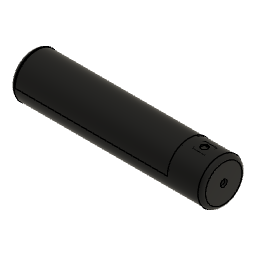
Laser_Pointer_Assembled (Autodesk Fusion 360 archive; units mm, degrees)
design "Laser_Pointer_Case"
Autodesk Fusion 360 part; units mm, degrees
sketch "Sketch1" plane through (0, 0, 0) normal (1, 0, 0) x (0, 1, 0)
  circle A0 centre (0, 0) radius 9.5
  circle A1 centre (0, 0) radius 11.5
  dimension "d1" = 19
  dimension "d2" = 23
  constraint coincident A0.centre A1.centre
  measures "d1" diameter of A0
  measures "d2" diameter of A1
extrude "Extrude1" add sketch "Sketch1" along normal blind 50 makes body 1
extrude "Extrude2" add 1 faces at (0, 10.7551, -1.0433) along direction (-1, 0, 0) blind 50 on bodies 1 bodies 1
sketch "Sketch3" plane through (-50, 0, 0) normal (-1, 0, 0) x (0, -1, 0)
  circle A0 centre (0, 0) radius 9.5
  circle A1 centre (0, 0) radius 11.5
extrude "Extrude4" add sketch "Sketch3" against normal blind 5 contours A0 bodies 1
ref_plane "WorkPlane1" through (0, 0, -11.5) normal (0, 0, 1) x (1, 0, 0)
sketch "Sketch2" plane through (0, 0, -11.5) normal (0, 0, 1) x (1, 0, 0)
  line L0 (-45, -15.7965) -> (35, -15.7965)
  line L1 (35, -15.7965) -> (35, 17.9404)
  line L2 (35, 17.9404) -> (-45, 17.9404)
  line L3 (-45, 17.9404) -> (-45, -15.7965)
  circle A0 through (-50, 11.5, 11.5) (-50, -5.75, 21.4593) (-50, -5.75, 1.5407)
  point P0 (-50, 0)
  dimension "d8" = 80
  dimension "d16" = 5
  constraint horizontal L0
  constraint vertical L1
  constraint horizontal L2
  constraint vertical L3
  measures "d8" distance of L0.start L0.end
  measures "d16" distance of L3 P0
extrude "Extrude3" cut sketch "Sketch2" along normal blind 11.5 bodies 1
sketch "Sketch4" plane through (35, 0, 0) normal (-1, 0, 0) x (0, -1, 0)
  arc A0 (-9.5, 0) -> (9.5, 0) centre (0, 0) ccw
  line L0 (-9.5, 0) -> (-11.5, 0)
  arc A1 (-11.5, 0) -> (11.5, 0) centre (0, 0) ccw
  line L1 (11.5, 0) -> (9.5, 0)
  circle A2 centre (0, 0) radius 9.5
  dimension "d13" = 19
  constraint coincident A0.centre A1.centre
  measures "d13" diameter of A2
extrude "Extrude5" add sketch "Sketch4" against normal blind 2 contours A0 A2 bodies 1
sketch "Sketch5" plane through (-45, 0, 0) normal (1, 0, 0) x (0, 1, 0)
  arc A0 (9.5, 0) -> (-9.5, 0) centre (0, 0) ccw
  line L0 (-9.5, 0) -> (-11.5, 0)
  arc A1 (-11.5, 0) -> (11.5, 0) centre (0, 0) ccw
  line L1 (11.5, 0) -> (9.5, 0)
  circle A2 centre (0, 0) radius 9.5
  dimension "d17" = 19
  constraint coincident A0.centre A1.centre
  measures "d17" diameter of A2
extrude "Extrude6" add sketch "Sketch5" along normal blind 80 separate body contours L0 A1 L1 A2 makes body 2
extrude "Extrude7" cut 1 faces at (-45, -0.2865, -3.8226) along direction (-1, 0, 0) blind 2.5 on bodies 1 bodies 1
extrude "Extrude8" add 1 faces at (-45, 10.5848, -2.1732) along direction (-1, 0, 0) blind 2.5 on bodies 2 bodies 2
sketch "Sketch6" plane through (-47.5, 0, 0) normal (-1, 0, 0) x (0, -1, 0)
  line L0 (11.5, 0) -> (9.5, 0)
  arc A0 (-9.5, 0) -> (9.5, 0) centre (0, 0) ccw
  line L1 (-9.5, 0) -> (-11.5, 0)
  arc A1 (-11.5, 0) -> (11.5, 0) centre (0, 0) ccw
  circle A2 centre (0, 0) radius 9.5
  dimension "d24" = 19
  constraint concentric A0 A2
  measures "d24" diameter of A2
extrude "Extrude9" add sketch "Sketch6" against normal blind 2.5 contours A0 A2 bodies 2
sketch "Sketch7" plane through (-50, 0, 0) normal (-1, 0, 0) x (0, -1, 0)
  circle A0 centre (0, 0) radius 11.5
  circle A1 centre (0, 0) radius 1.25
  dimension "d27" = 2.5
  constraint concentric A0 A1
  measures "d27" diameter of A1
extrude "Extrude10" cut sketch "Sketch7" against normal blind 5 contours A1 bodies 1 2
ref_plane "WorkPlane2" through (-39.5, 0, -1) normal (1, 0, 0) x (0, 1, 0)
sketch "Sketch8" plane through (-39.5, 0, 0) normal (1, 0, 0) x (0, 1, 0)
  circle A0 centre (0, 0) radius 9.5
  dimension "d31" = 19
  constraint coincident A0.centre origin
  measures "d31" diameter of A0
extrude "Extrude11" add sketch "Sketch8" along normal blind 2 bodies 1
sketch "Sketch9" plane through (35, 0, 0) normal (-1, 0, 0) x (0, -1, 0)
  line L0 (-9.5, 0) -> (-11.5, 0)
  arc A0 (-11.5, 0) -> (11.5, 0) centre (0, 0) ccw
  line L1 (11.5, 0) -> (9.5, 0)
  arc A1 (9.5, 0) -> (-9.5, 0) centre (0, 0) ccw
  circle A2 centre (0, 0) radius 2.5
  dimension "d34" = 5
  constraint coincident A0.centre A1.centre
  measures "d34" diameter of A2
extrude "Extrude12" cut sketch "Sketch9" against normal blind 2 contours A2 bodies 1
sketch "Sketch10" plane through (-37.5, 0, 0) normal (1, 0, 0) x (0, 1, 0)
  arc A0 (-9.5, 0) -> (9.5, 0) centre (0, 0) ccw
  arc A1 (9.5, 0) -> (-9.5, 0) centre (0, 0) ccw
  circle A2 centre (0, 0) radius 2.5
  dimension "d37" = 5
  constraint coincident A0.centre A1.centre
  measures "d37" diameter of A2
extrude "Extrude13" cut sketch "Sketch10" against normal blind 2 contours A2 bodies 1
extrude "Extrude14" add 1 faces at (35, -7.3712, -2.0248) along direction (-1, 0, 0) blind 3 on bodies 1 bodies 1
extrude "Extrude15" cut 1 faces at (37, 7.122, 0.5962) along direction (-1, 0, 0) blind 4 on bodies 1 bodies 1
extrude "Extrude16" cut 1 faces at (50, 10.7551, -1.0433) along direction (-1, 0, 0) blind 2 on bodies 1 bodies 1
sketch "Sketch11" plane through (48, 0, 0) normal (1, 0, 0) x (0, 1, 0)
  circle A0 centre (0, 0) radius 9.5
  circle A1 centre (0, 0) radius 11.5
  circle A2 centre (0, 0) radius 11.5
  dimension "d46" = 23
  constraint concentric A0 A2
  measures "d46" diameter of A2
extrude "Extrude17" add sketch "Sketch11" along normal blind 2 separate body contours A0 | A1 A2 makes body 3
sketch "Sketch12" plane through (50, 0, 0) normal (1, 0, 0) x (0, 1, 0)
  circle A0 centre (0, 0) radius 11.5
  circle A1 centre (0, 0) radius 1.75
  dimension "d49" = 3.5
  constraint coincident A0.centre A1.centre
  measures "d49" diameter of A1
extrude "Extrude18" cut sketch "Sketch12" against normal blind 2 contours A1 bodies 3
sketch "Sketch13" plane through (48, 0, 0) normal (1, 0, 0) x (0, 1, 0)
  circle A0 centre (0, 0) radius 9.5
  circle A1 centre (0, 0) radius 11.5
  circle A2 centre (0, 0) radius 10.875
  circle A3 centre (0, 0) radius 10.125
  circle A4 centre (0, 0) radius 10.925
  circle A5 centre (0, 0) radius 10.075
  dimension "d52" = 21.75
  dimension "d53" = 20.25
  dimension "d54" = 0.05
  dimension "d55" = -0.05
  constraint concentric A0 A2
  constraint concentric A0 A3
  measures "d52" diameter of A2
  measures "d53" diameter of A3
extrude "Extrude19" cut sketch "Sketch13" against normal blind 3 contours A2 | A3 | A4 bodies 1
sketch "Sketch14" plane through (48, 0, 0) normal (-1, 0, 0) x (0, -1, 0)
  circle A0 centre (0, 0) radius 1.75
  circle A1 centre (0, 0) radius 11.5
  circle A2 centre (0, -0.0586) radius 3
  circle A3 centre (0, -0.0586) radius 3.2
  circle A4 centre (0, 0) radius 10.925
  circle A5 centre (0, 0) radius 10.075
  circle A6 centre (0, 0) radius 10.875
  circle A7 centre (0, 0) radius 10.125
  dimension "d58" = 0.2
  dimension "d61" = -0.05
  dimension "d62" = 0.05
extrude "Extrude20" cut sketch "Sketch14" against normal blind 0.75 contours A2 | A3 bodies 3
extrude "Extrude21" add sketch "Sketch14" along normal blind 2.9 contours A6 bodies 3
ref_plane "WorkPlane3" through (0, 0, 9) normal (0, 0, 1) x (1, 0, 0)
ref_plane "WorkPlane4" through (0, 0, -11.5) normal (0, 0, 1) x (1, 0, 0)
sketch "Sketch17" plane through (0, 0, -11.5) normal (0, 0, 1) x (1, 0, 0)
  circle A0 centre (40, 0) radius 1.75
  dimension "d76" = 3.5
  measures "d76" diameter of A0
extrude "Extrude24" cut sketch "Sketch17" along normal blind 2.5 bodies 1
ref_plane "WorkPlane5" through (0, 0, -8.5) normal (0, 0, 1) x (1, 0, 0)
sketch "Sketch18" plane through (0, 0, -8.5) normal (0, 0, 1) x (1, 0, 0)
  line L0 (42.9931, -3) -> (36.9931, -3)
  line L1 (42.9931, 3) -> (42.9931, -3)
  line L2 (36.9931, -3) -> (36.9931, 3)
  line L3 (36.9931, 3) -> (42.9931, 3)
  line L4 (43.1931, 3.2) -> (43.1931, -3.2)
  line L5 (43.1931, -3.2) -> (36.7931, -3.2)
  line L6 (36.7931, -3.2) -> (36.7931, 3.2)
  line L7 (36.7931, 3.2) -> (43.1931, 3.2)
  dimension "d80" = -0.2
extrude "Extrude25" cut sketch "Sketch18" against normal blind 2.3 contours L0 L1 L2 L3 | L4 L5 L6 L7 bodies 1
fillet "Fillet1" radius 2 2 edges at (-50, -10.7218, 4.1586) (50, -10.7218, -4.1586) on bodies 1 3
sketch "Sketch19" plane through (-37.5, 0, 0) normal (1, 0, 0) x (0, 1, 0)
  circle A0 centre (0, 0) radius 2.5
  arc A1 (-9.5, 0) -> (9.5, 0) centre (0, 0) ccw
  arc A2 (9.5, 0) -> (-9.5, 0) centre (0, 0) ccw
  circle A3 centre (0, 0) radius 4
  dimension "d85" = 8
  constraint concentric A0 A3
  measures "d85" diameter of A3
extrude "Extrude26" cut sketch "Sketch19" against normal blind 0.5 contours A3 bodies 1
sketch "Sketch20" plane through (32, 0, 0) normal (-1, 0, 0) x (0, -1, 0)
  circle A0 centre (0, 0) radius 2.5
  line L0 (-9.5, 0) -> (-11.5, 0)
  arc A1 (-11.5, 0) -> (11.5, 0) centre (0, 0) ccw
  line L1 (11.5, 0) -> (9.5, 0)
  arc A2 (9.5, 0) -> (-9.5, 0) centre (0, 0) ccw
  circle A3 centre (0, 0) radius 4
  dimension "d88" = 8
  constraint coincident A0.centre A1.centre
  measures "d88" diameter of A3
extrude "Extrude29" cut 1 faces at (35, 10.5848, -2.1732) along direction (-1, 0, 0) blind 3 on bodies 2 bodies 2
sketch "Sketch21" plane through (32, 0, 0) normal (1, 0, 0) x (0, 1, 0)
  line L0 (-9.5, 0) -> (-11.5, 0)
  arc A0 (-11.5, 0) -> (11.5, 0) centre (0, 0) ccw
  line L1 (11.5, 0) -> (9.5, 0)
  arc A1 (-9.5, 0) -> (9.5, 0) centre (0, 0) ccw
  circle A2 centre (0, 0) radius 10.875
  circle A3 centre (0, 0) radius 10.125
  line L2 (10.8638, -0.4934) -> (10.113, -0.4934)
  line L3 (-10.113, -0.4935) -> (-10.8638, -0.4935)
  line L4 (0, -10.875) -> (0, -10.125)
  line L5 (0, 0) -> (7.6898, -7.6898)
  line L6 (0, 0) -> (10.875, 0) construction
  line L7 (0, 0) -> (-7.6898, -7.6898)
  line L8 (0, 0) -> (-4.1617, -10.0472)
  line L9 (0, 0) -> (10.875, 0) construction
  line L10 (0, 0) -> (4.1617, -10.0472)
  line L11 (0, 0) -> (-10.0472, -4.1617)
  line L12 (0, 0) -> (10.875, 0) construction
  line L13 (0, 0) -> (10.0472, -4.1617)
  line L14 (-9.5, 0) -> (-11.5, 0)
  arc A4 (-11.5, 0) -> (11.5, 0) centre (0, 0) ccw
  line L15 (11.5, 0) -> (9.5, 0)
  arc A5 (-9.5, 0) -> (9.5, 0) centre (0, 0) ccw
  dimension "d91" = 21.75
  dimension "d92" = 20.25
  dimension "d93" = 45
  dimension "d94" = 90
  dimension "d95" = 112.5
  dimension "d96" = 157.5
  constraint concentric A0 A2
  constraint concentric A2 A3
  constraint coincident A2 L2.start
  constraint coincident A3 L2.end
  constraint horizontal L2
  constraint coincident A3 L3.start
  constraint coincident A2 L3.end
  constraint parallel L2 L3
  constraint coincident A2 L4.start
  constraint coincident A3 L4.end
  constraint vertical L4
  constraint horizontal L6
  constraint coincident A0.centre A1.centre
  constraint coincident A2 L5.end
  constraint coincident A2 L7.end
  constraint horizontal L9
  constraint coincident A2 L8.end
  constraint coincident A2 L10.end
  constraint horizontal L12
  constraint coincident A2 L11.end
  constraint coincident A2 L13.end
  constraint perpendicular L8 L13
  measures "d91" diameter of A2
  measures "d92" diameter of A3
  measures "d93" angle of L5 L6
  measures "d94" angle of L5 L7
  measures "d95" angle of L8 L9
  measures "d96" angle of L11 L12
extrude "Extrude28" add sketch "Sketch21" along normal blind 0.5 contours A2 A3 L3 L11 | A2 A3 L2 L13 | A2 A3 L7 L8 | A2 A3 L5 L10 bodies 2
sketch "Sketch22" plane through (32, 0, 0) normal (-1, 0, 0) x (0, -1, 0)
  circle A0 centre (0, 0) radius 2.5
  line L0 (-9.5, 0) -> (-11.5, 0)
  arc A1 (-11.5, 0) -> (11.5, 0) centre (0, 0) ccw
  line L1 (11.5, 0) -> (9.5, 0)
  arc A2 (9.5, 0) -> (-9.5, 0) centre (0, 0) ccw
  line L2 (-3.8747, -9.3543) -> (-4.1617, -10.0472)
  arc A3 (-7.6898, -7.6898) -> (-4.1617, -10.0472) centre (0, 0) ccw
  line L3 (-7.6898, -7.6898) -> (-7.1595, -7.1595)
  arc A4 (-7.1595, -7.1595) -> (-3.8747, -9.3543) centre (0, 0) ccw
  line L4 (-9.3543, -3.8747) -> (-10.0472, -4.1617)
  arc A5 (-10.8638, -0.4934) -> (-10.0472, -4.1617) centre (0, 0) ccw
  line L5 (-10.8638, -0.4934) -> (-10.113, -0.4934)
  arc A6 (-10.113, -0.4934) -> (-9.3543, -3.8747) centre (0, 0) ccw
  arc A7 (4.1617, -10.0472) -> (7.6898, -7.6898) centre (0, 0) ccw
  line L6 (4.1617, -10.0472) -> (3.8747, -9.3543)
  arc A8 (3.8747, -9.3543) -> (7.1595, -7.1595) centre (0, 0) ccw
  line L7 (7.1595, -7.1595) -> (7.6898, -7.6898)
  arc A9 (10.0472, -4.1617) -> (10.8638, -0.4935) centre (0, 0) ccw
  line L8 (10.0472, -4.1617) -> (9.3543, -3.8747)
  arc A10 (9.3543, -3.8747) -> (10.113, -0.4935) centre (0, 0) ccw
  line L9 (10.113, -0.4935) -> (10.8638, -0.4935)
  line L10 (7.158, -6.8752) -> (7.9714, -7.6885)
  arc A11 (4.0528, -10.3068) -> (7.9714, -7.6885) centre (0, 0) ccw
  line L11 (4.0528, -10.3068) -> (3.6126, -9.2442)
  arc A12 (3.6126, -9.2442) -> (7.158, -6.8752) centre (0, 0) ccw
  line L12 (9.9207, -0.2935) -> (11.0711, -0.2935)
  arc A13 (10.1538, -4.4223) -> (11.0711, -0.2935) centre (0, 0) ccw
  line L13 (10.1538, -4.4223) -> (9.0911, -3.9821)
  arc A14 (9.0911, -3.9821) -> (9.9207, -0.2935) centre (0, 0) ccw
  line L14 (-3.6126, -9.2442) -> (-4.0528, -10.3068)
  arc A15 (-7.9714, -7.6885) -> (-4.0528, -10.3068) centre (0, 0) ccw
  line L15 (-7.9714, -7.6885) -> (-7.158, -6.8752)
  arc A16 (-7.158, -6.8752) -> (-3.6126, -9.2442) centre (0, 0) ccw
  line L16 (-9.0911, -3.9821) -> (-10.1538, -4.4223)
  arc A17 (-11.0711, -0.2934) -> (-10.1538, -4.4223) centre (0, 0) ccw
  line L17 (-11.0711, -0.2934) -> (-9.9207, -0.2934)
  arc A18 (-9.9207, -0.2934) -> (-9.0911, -3.9821) centre (0, 0) ccw
  dimension "d101" = 0.2
  dimension "d102" = -0.2
  dimension "d103" = 0.2
  dimension "d104" = 0.2
extrude "Extrude30" cut sketch "Sketch22" against normal blind 0.6 contours L2 A3 L3 A4 | L4 A5 L5 A6 | A7 L6 A8 L7 | A9 L8 A10 L9 | L10 A11 L11 A12 | L12 A13 L13 A14 | L14 A15 L15 A16 | L16 A17 L17 A18 bodies 1
extrude "Extrude27" cut sketch "Sketch20" against normal blind 0.2 contours A3 bodies 1
sketch "Sketch23" plane through (33, 0, 0) normal (1, 0, 0) x (0, 1, 0)
  circle A0 centre (0, 0) radius 2.5
  circle A1 centre (0, 0) radius 9.5
  circle A2 centre (0.0005, 9.5) radius 1.425
  dimension "d108" = 2.85
  constraint coincident A1 A2.centre
  measures "d108" diameter of A2
extrude "Extrude31" cut sketch "Sketch23" against normal blind 80.5 contours A1 A2 | A1 A2 picked at (0.0005, 9.0171) picked at (-0.0173, 9.9667) bodies 1
extrude "Extrude32" cut 1 faces at (33, -0.0173, 9.9667) along direction (1, 0, 0) blind 15 on bodies 1 bodies 1
move_body "Move1" bodies 2 1 3 to x (1, 0, 0) y (0, -1, 0) z (0, 0, -1) at (0, 0, 0)
named bodies: "Body", "SideCap", "FrontCap"

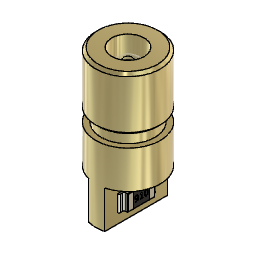
design "Laser_5mW"
Autodesk Fusion 360 part; units mm, degrees
sketch "Sketch1" plane through (0, 0, 0) normal (0, 0, 1) x (1, 0, 0)
  circle A0 centre (0, 0) radius 3
  dimension "d1" = 6
  constraint coincident A0.centre origin
  measures "d1" diameter of A0
extrude "Extrude1" add sketch "Sketch1" along normal blind 7 makes body 1
sketch "Sketch2" plane through (0, 0, 7) normal (0, 0, 1) x (-1, 0, 0)
  circle A0 centre (0, 0) radius 3
  circle A1 centre (0, 0) radius 2.5
  dimension "d4" = 5
  constraint concentric A0 A1
  measures "d4" diameter of A1
extrude "Extrude2" add sketch "Sketch2" along normal blind 1 contours A1 bodies 1
sketch "Sketch3" plane through (0, 0, 8) normal (0, 0, 1) x (-1, 0, 0)
  circle A0 centre (0, 0) radius 2.5
  circle A1 centre (0, 0) radius 3
  dimension "d7" = 6
  constraint concentric A0 A1
  measures "d7" diameter of A1
extrude "Extrude3" add sketch "Sketch3" along normal blind 5 contours A0 | A1 bodies 1
sketch "Sketch4" plane through (0, 0, 0) normal (0, 0, -1) x (1, 0, 0)
  circle A0 centre (0, 0) radius 3
  line L0 (-0.75, 2.9047) -> (-0.75, -2.9047)
  line L1 (0.75, 2.9047) -> (0.75, -2.9047)
  dimension "d10" = 0.75
  dimension "d11" = 0.75
  constraint coincident A0 L0.start
  constraint coincident A0 L0.end
  constraint vertical L0
  constraint coincident A0 L1.start
  constraint coincident A0 L1.end
  constraint parallel L0 L1
  measures "d10" distance of A0.centre L0
  measures "d11" distance of A0.centre L1
extrude "Extrude4" cut sketch "Sketch4" against normal blind 3.5 contours A0 L1 | A0 L0 bodies 1
sketch "Sketch5" plane through (0, 0, 13) normal (0, 0, 1) x (-1, 0, 0)
  circle A0 centre (0, 0) radius 3
  circle A1 centre (0, 0) radius 1.5
  dimension "d14" = 3
  constraint coincident A0.centre A1.centre
  measures "d14" diameter of A1
extrude "Extrude5" cut sketch "Sketch5" against normal blind 3 contours A1 bodies 1
sketch "Sketch6" plane through (0, 0, 10) normal (0, 0, 1) x (-1, 0, 0)
  circle A0 centre (0, 0) radius 1.5
  circle A1 centre (0, 0) radius 1.4
  dimension "d17" = 2.8
  constraint concentric A0 A1
  measures "d17" diameter of A1
extrude "Extrude6" add sketch "Sketch6" along normal blind 2 separate body contours A1 makes body 2
fillet "Fillet1" radius 1 1 edges at (1.3053, 0.5063, 12) on bodies 2
chamfer "Chamfer1" distance 0.25 angle 45 2 edges at (2.797, 1.0848, 13) (2.797, 1.0848, 8) on bodies 1
sketch "Sketch7" plane through (-0.75, 0, 0) normal (-1, 0, 0) x (0, -1, 0)
  line L0 (-2.9047, 0) -> (2.9047, 0)
  line L1 (2.9047, 0) -> (2.9047, 3.5)
  line L2 (2.9047, 3.5) -> (-2.9047, 3.5)
  line L3 (-2.9047, 3.5) -> (-2.9047, 0)
  circle A0 centre (0, 1.6) radius 1
  dimension "d23" = 2
  measures "d23" diameter of A0
extrude "Extrude7" add sketch "Sketch7" along normal blind 0.5 contours A0 bodies 1
fillet "Fillet2" radius 0.75 1 edges at (-1.25, 0.9323, 1.2384) on bodies 1
sketch "Sketch8" plane through (0.75, 0, 0) normal (1, 0, 0) x (0, 1, 0)
  line L0 (-2.9047, 0) -> (2.9047, 0)
  line L1 (2.9047, 0) -> (2.9047, 3.5)
  line L2 (2.9047, 3.5) -> (-2.9047, 3.5)
  line L3 (-2.9047, 3.5) -> (-2.9047, 0)
  line L4 (1.75, 0.9391) -> (-1.75, 0.9391)
  line L5 (-1.75, 0.9391) -> (-1.75, 2.4391)
  line L6 (-1.75, 2.4391) -> (1.75, 2.4391)
  line L7 (1.75, 2.4391) -> (1.75, 0.9391)
  line L8 (1.75, 0.9391) -> (-1.75, 2.4391) construction
  line L9 (-1.75, 0.9391) -> (1.75, 2.4391) construction
  line L10 (-1.75, 2.4391) -> (-1.25, 2.4391)
  line L11 (-1.25, 2.4391) -> (-1.25, 0.9391)
  line L12 (-1.25, 0.9391) -> (-1.75, 0.9391)
  line L13 (-1.75, 0.9391) -> (-1.75, 2.4391)
  line L14 (1.75, 2.4391) -> (1.25, 2.4391)
  line L15 (1.25, 2.4391) -> (1.25, 0.9391)
  line L16 (1.25, 0.9391) -> (1.75, 0.9391)
  line L17 (1.75, 0.9391) -> (1.75, 2.4391)
  line L18 (-1.25, 2.4391) -> (-0.75, 2.4391)
  line L19 (-0.75, 2.4391) -> (-0.75, 0.9391)
  line L20 (-0.75, 0.9391) -> (-1.25, 0.9391)
  line L21 (-1.25, 0.9391) -> (-1.25, 2.4391)
  line L22 (1.25, 2.4391) -> (0.75, 2.4391)
  line L23 (0.75, 2.4391) -> (0.75, 0.9391)
  line L24 (0.75, 0.9391) -> (1.25, 0.9391)
  line L25 (1.25, 0.9391) -> (1.25, 2.4391)
  point P0 (0, 1.6891)
  dimension "d28" = 3.5
  dimension "d29" = 1.5
  dimension "d30" = 0.5
  dimension "d31" = 1.5
  dimension "d32" = 0.5
  dimension "d33" = 0.5
  dimension "d34" = 0.5
  constraint horizontal L4
  constraint perpendicular L4 L5
  constraint parallel L4 L6
  constraint parallel L5 L7
  constraint coincident L8 P0
  constraint coincident L9 P0
  constraint horizontal L10
  constraint vertical L11
  constraint horizontal L12
  constraint vertical L13
  constraint horizontal L14
  constraint vertical L15
  constraint horizontal L16
  constraint vertical L17
  constraint coincident L4 L15.end
  constraint horizontal L18
  constraint vertical L19
  constraint horizontal L20
  constraint vertical L21
  constraint coincident L4 L19.end
  constraint horizontal L22
  constraint vertical L23
  constraint horizontal L24
  constraint vertical L25
  constraint coincident L4 L23.end
  measures "d28" distance of L5.end L6.end
  measures "d29" distance of L4.end L5.end
  measures "d30" distance of L5.end L10.end
  measures "d31" distance of L5.end L4.end
  measures "d32" distance of L6.end L14.end
  measures "d33" distance of L10.end L18.end
  measures "d34" distance of L14.end L22.end
extrude "Extrude8" add sketch "Sketch8" along normal blind 0.15 contours L4 L6 L7 L14 L15 L16 L17 L25 | L4 L5 L6 L10 L11 L12 L13 L21 bodies 1
extrude "Extrude9" add sketch "Sketch8" along normal blind 0.5 contours L4 L6 L15 L22 L23 L24 L25 | L4 L6 L11 L18 L19 L20 L21 bodies 1
extrude "Extrude10" add sketch "Sketch8" along normal blind 0.5 separate body contours L4 L6 L19 L23 makes body 3
fillet "Fillet3" radius 0.15 4 edges at (0.9, -1.75, 1.6891) (0.9, 1.75, 1.6891) (0.9, -1.25, 1.6891) (0.9, 1.25, 1.6891) on bodies 1 3
fillet "Fillet3" radius 0.05 8 edges at (1.25, 1.25, 1.6891) (1.25, 1, 0.9391) (1.25, -1, 0.9391) (1.25, -1.25, 1.6891) (1.25, -1, 2.4391) (1.25, 1, 2.4391) (1.25, 0, 0.9391) (1.25, 0, 2.4391) on bodies 1 3
sketch "Sketch9" plane through (1.25, 0, 0) normal (1, 0, 0) x (0, 1, 0)
  line L0 (0.75, 2.3891) -> (-0.75, 2.3891)
  line L1 (-0.75, 2.3891) -> (-0.75, 0.9891)
  line L2 (-0.75, 0.9891) -> (0.75, 0.9891)
  line L3 (0.75, 0.9891) -> (0.75, 2.3891)
  line L4 (-0.5459, 1.3459) -> (0.5541, 1.3459) construction
  line L5 (0.5541, 1.3459) -> (0.5541, 2.0459) construction
  line L6 (0.5541, 2.0459) -> (-0.5459, 2.0459) construction
  line L7 (-0.5459, 2.0459) -> (-0.5459, 1.3459) construction
  dimension "d45" = 0.5
  text T0 "910" font "Verdana" height 0.5 align centre middle in box 1.1 x 0.7 at (-0.5459, 1.3459) x (1, 0) y (0, 1) spacing 1 kerned
extrude "Extrude11" add sketch "Sketch9" along normal blind 0.005 text T0 bodies 3
